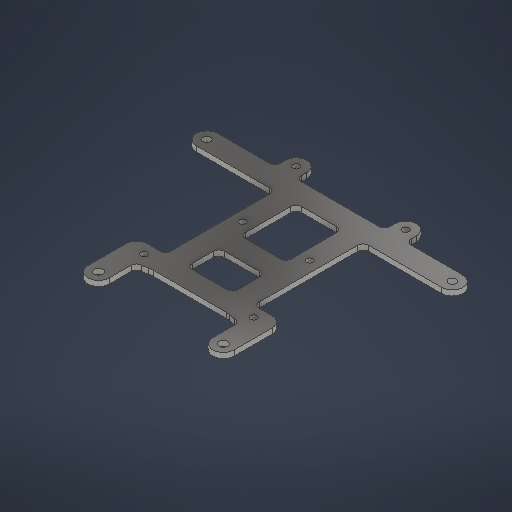
# Autodesk Inventor part: Trägerblech
Saved by Autodesk Inventor 2025.2 (Build 292293000, 293)
## iProperties
Created: 2024-12-09
Part Number: Trägerblech
Material: Generisch
Document SubType Name: Modeling
Designer: Fabian
Density: 1 g/cm^3
Appearance: Stahl - poliert
Author: Fabian
Autodesk Inventor part; units mm, degrees
ref_plane "YZ Plane" through (0, 0, 0) normal (1, 0, 0) x (0, 1, 0)
ref_plane "XZ Plane" through (0, 0, 0) normal (0, 1, 0) x (-1, 0, 0)
ref_plane "XY Plane" through (0, 0, 0) normal (0, 0, 1) x (1, 0, 0)
sketch "Skizze1" plane through (0, 0, 0) normal (0, 1, 0) x (-1, 0, 0)
  circle A0 centre (30.623, -39.877) radius 2.1
  circle A1 centre (30.623, -39.877) radius 2.1
  circle A2 centre (46, -38.5) radius 1.85
  circle A3 centre (46, -38.5) radius 1.85
  circle A4 centre (-30.623, -39.877) radius 2.1
  circle A5 centre (-30.623, -39.877) radius 2.1
  circle A6 centre (-46, -38.5) radius 1.85
  circle A7 centre (-46, -38.5) radius 1.85
  circle A8 centre (-46, 19.5) radius 1.85
  circle A9 centre (-46, 19.5) radius 1.85
  circle A10 centre (-30.1839, 17.0814) radius 2.1
  circle A11 centre (-30.1839, 17.0814) radius 2.1
  circle A12 centre (30.1839, 17.0814) radius 2.1
  circle A13 centre (30.1839, 17.0814) radius 2.1
  circle A14 centre (46, 19.5) radius 1.85
  circle A15 centre (46, 19.5) radius 1.85
  circle A16 centre (23.4, 24.7201) radius 1.2779
  circle A17 centre (-23.4, 24.7201) radius 1.25
  arc A18 (-50, -38.5) -> (-46, -42.5) centre (-46, -38.5) ccw
  line L0 (-50, -38.5) -> (-50, 32.5)
  arc A19 (-46, 36.5) -> (-50, 32.5) centre (-46, 32.5) ccw
  line L1 (-46, 36.5) -> (46, 36.5)
  arc A20 (50, 32.5) -> (46, 36.5) centre (46, 32.5) ccw
  line L2 (50, 32.5) -> (50, -38.5)
  arc A21 (46, -42.5) -> (50, -38.5) centre (46, -38.5) ccw
  line L3 (46, -42.5) -> (36.4, -42.5)
  arc A22 (32.4, -38.5) -> (36.4, -42.5) centre (36.4, -38.5) ccw
  line L4 (32.4, -38.5) -> (32.4, -3.51)
  arc A23 (32.4, -3.51) -> (30.4, -1.51) centre (30.4, -3.51) ccw
  line L5 (30.4, -1.51) -> (-26.4, -1.51)
  arc A24 (-26.4, -1.51) -> (-28.4, -3.51) centre (-26.4, -3.51) ccw
  line L6 (-28.4, -3.51) -> (-28.4, -38.5)
  arc A25 (-32.4, -42.5) -> (-28.4, -38.5) centre (-32.4, -38.5) ccw
  line L7 (-32.4, -42.5) -> (-46, -42.5)
  circle A26 centre (-46, -38.5) radius 1.375
  circle A27 centre (46, 19.5) radius 1.375
  circle A28 centre (46, -38.5) radius 1.375
  circle A29 centre (-46, 19.5) radius 1.375
  line L8 (50, -42.5) -> (-50, -42.5)
  line L9 (-50, -42.5) -> (-50, 36.5)
  line L10 (-50, 36.5) -> (50, 36.5)
  line L11 (50, 36.5) -> (50, -42.5)
  circle A30 centre (-12.55, 10.5) radius 1
  circle A31 centre (-0.05, 10.5) radius 1
  circle A32 centre (-0.05, -10.5) radius 1
  circle A33 centre (-12.55, -10.5) radius 1
  line L12 (-12.55, 12.5) -> (7.45, 12.5)
  arc A34 (9.45, 10.5) -> (7.45, 12.5) centre (7.45, 10.5) ccw
  line L13 (9.45, 10.5) -> (9.45, -10.5)
  arc A35 (7.45, -12.5) -> (9.45, -10.5) centre (7.45, -10.5) ccw
  line L14 (7.45, -12.5) -> (-12.55, -12.5)
  arc A36 (-14.55, -10.5) -> (-12.55, -12.5) centre (-12.55, -10.5) ccw
  line L15 (-14.55, -10.5) -> (-14.55, 10.5)
  arc A37 (-12.55, 12.5) -> (-14.55, 10.5) centre (-12.55, 10.5) ccw
  line L16 (4.8641, 52.5092) -> (13.75, 52.5092)
  arc A38 (19.2723, 46.9869) -> (13.75, 52.5092) centre (13.75, 46.9869) ccw
  line L17 (19.2723, 46.9869) -> (19.2723, 29.5841)
  ellipse E0 centre (20.2732, 29.5863) end of major axis (19.6049, 28.8395) minor radius 1 (19.2723, 29.5841) -> (20.1839, 28.5889) ccw
  line L18 (20.1839, 28.5889) -> (23.7114, 28.2803)
  arc A39 (23.7114, 21.1599) -> (23.7114, 28.2803) centre (23.4, 24.7201) ccw
  line L19 (23.7114, 21.1599) -> (20.1839, 20.8513)
  ellipse E1 centre (20.2732, 19.8539) end of major axis (19.6049, 20.6006) minor radius 1 (20.1839, 20.8513) -> (19.2723, 19.856) ccw
  line L20 (19.2723, 19.856) -> (19.2723, 19.487)
  arc A40 (13.75, 13.9647) -> (19.2723, 19.487) centre (13.75, 19.487) ccw
  line L21 (13.75, 13.9647) -> (-13.75, 13.9647)
  arc A41 (-19.2723, 19.487) -> (-13.75, 13.9647) centre (-13.75, 19.487) ccw
  line L22 (-19.2723, 19.487) -> (-19.2723, 19.856)
  ellipse E2 centre (-20.2732, 19.8539) end of major axis (-19.6049, 20.6006) minor radius 1 (-19.2723, 19.856) -> (-20.1839, 20.8513) ccw
  line L23 (-20.1839, 20.8513) -> (-23.7114, 21.1599)
  arc A42 (-23.7114, 28.2803) -> (-23.7114, 21.1599) centre (-23.4, 24.7201) ccw
  line L24 (-23.7114, 28.2803) -> (-20.1839, 28.5889)
  ellipse E3 centre (-20.2732, 29.5863) end of major axis (-19.6049, 28.8395) minor radius 1 (-20.1839, 28.5889) -> (-19.2723, 29.5841) ccw
  line L25 (-19.2723, 29.5841) -> (-19.2723, 46.9869)
  arc A43 (-13.75, 52.5092) -> (-19.2723, 46.9869) centre (-13.75, 46.9869) ccw
  line L26 (-13.75, 52.5092) -> (-4.8641, 52.5092)
  ellipse E4 centre (-4.8662, 53.5102) end of major axis (-4.1194, 52.8419) minor radius 1 (-4.8641, 52.5092) -> (-3.8688, 53.4208) ccw
  line L27 (-3.8688, 53.4208) -> (-3.5602, 56.9484)
  arc A44 (3.5602, 56.9484) -> (-3.5602, 56.9484) centre (0, 56.6369) ccw
  line L28 (3.5602, 56.9484) -> (3.8688, 53.4208)
  ellipse E5 centre (4.8662, 53.5102) end of major axis (4.1194, 52.8419) minor radius 1 (3.8688, 53.4208) -> (4.8641, 52.5092) ccw
  line L29 (-12.55, -14.5) -> (7.45, -14.5)
  arc A45 (7.45, -14.5) -> (11.45, -10.5) centre (7.45, -10.5) ccw
  line L30 (11.45, -10.5) -> (11.45, 10.5)
  arc A46 (11.45, 10.5) -> (7.45, 14.5) centre (7.45, 10.5) ccw
  line L31 (7.45, 14.5) -> (-12.55, 14.5)
  arc A47 (-12.55, 14.5) -> (-16.55, 10.5) centre (-12.55, 10.5) ccw
  line L32 (-16.55, 10.5) -> (-16.55, -10.5)
  arc A48 (-16.55, -10.5) -> (-12.55, -14.5) centre (-12.55, -10.5) ccw
  line L33 (-12.55, -12.7) -> (7.45, -12.7)
  arc A49 (7.45, -12.7) -> (9.65, -10.5) centre (7.45, -10.5) ccw
  line L34 (9.65, -10.5) -> (9.65, 10.5)
  arc A50 (9.65, 10.5) -> (7.45, 12.7) centre (7.45, 10.5) ccw
  line L35 (7.45, 12.7) -> (-12.55, 12.7)
  arc A51 (-12.55, 12.7) -> (-14.75, 10.5) centre (-12.55, 10.5) ccw
  line L36 (-14.75, 10.5) -> (-14.75, -10.5)
  arc A52 (-14.75, -10.5) -> (-12.55, -12.7) centre (-12.55, -10.5) ccw
  line L37 (16.55, 14.5) -> (-16.55, 14.5)
  line L38 (-16.55, 14.5) -> (-16.55, -14.5)
  line L39 (-16.55, -14.5) -> (16.55, -14.5)
  line L40 (16.55, -14.5) -> (16.55, 14.5)
  line L41 (16.55, 14.5) -> (-16.55, -14.5) construction
  line L42 (-16.55, 14.5) -> (16.55, -14.5) construction
  line L43 (16.55, -14.5) -> (8.55, -14.5)
  line L44 (12.55, -14.5) -> (12.55, -9.5)
  line L45 (16.55, 14.5) -> (16.55, 6.5)
  line L46 (16.55, 10.5) -> (12.55, 10.5)
  line L47 (23.4, 24.7201) -> (23.4, 10.5)
  line L48 (12.55, 10.5) -> (23.4, 10.5) construction
  line L49 (12.55, 14.5) -> (23.4, 14.5)
  line L50 (23.4, 6.5) -> (12.55, 6.5)
  arc A53 (12.55, 14.5) -> (12.55, 6.5) centre (12.55, 10.5) ccw
  arc A54 (23.4, 6.5) -> (23.4, 14.5) centre (23.4, 10.5) ccw
  line L51 (23.4, 10.5) -> (23.4, 24.7201) construction
  line L52 (19.4, 10.5) -> (19.4, 24.7201)
  line L53 (27.4, 24.7201) -> (27.4, 10.5)
  arc A55 (19.4, 10.5) -> (27.4, 10.5) centre (23.4, 10.5) ccw
  arc A56 (27.4, 24.7201) -> (19.4, 24.7201) centre (23.4, 24.7201) ccw
  line L54 (0, -14.5) -> (0, 12.7) construction
  line L55 (12.55, -9.5) -> (12.55, -38.5) construction
  line L56 (8.55, -9.5) -> (8.55, -38.5)
  line L57 (16.55, -38.5) -> (16.55, -9.5)
  arc A57 (16.55, -9.5) -> (8.55, -9.5) centre (12.55, -9.5) ccw
  arc A58 (8.55, -38.5) -> (16.55, -38.5) centre (12.55, -38.5) ccw
  line L58 (12.55, -38.5) -> (46, -38.5) construction
  line L59 (12.55, -42.5) -> (46, -42.5)
  line L60 (46, -34.5) -> (12.55, -34.5)
  arc A59 (12.55, -34.5) -> (12.55, -42.5) centre (12.55, -38.5) ccw
  arc A60 (46, -42.5) -> (46, -34.5) centre (46, -38.5) ccw
  line L61 (-16.55, -14.5) -> (-8.55, -14.5)
  line L62 (-12.55, -14.5) -> (-12.55, -9.5)
  line L63 (-16.55, 14.5) -> (-16.55, 6.5)
  line L64 (-16.55, 10.5) -> (-12.55, 10.5)
  line L65 (-12.55, 10.5) -> (-23.4, 10.5) construction
  line L66 (-12.55, -9.5) -> (-12.55, -38.5) construction
  line L67 (-12.55, -9.5) -> (-12.55, -38.5) construction
  line L68 (-16.55, -9.5) -> (-16.55, -38.5)
  line L69 (-8.55, -38.5) -> (-8.55, -9.5)
  arc A61 (-8.55, -9.5) -> (-16.55, -9.5) centre (-12.55, -9.5) ccw
  arc A62 (-16.55, -38.5) -> (-8.55, -38.5) centre (-12.55, -38.5) ccw
  line L70 (-12.55, 10.5) -> (-23.4, 10.5) construction
  line L71 (-12.55, 14.5) -> (-23.4, 14.5)
  line L72 (-23.4, 6.5) -> (-12.55, 6.5)
  arc A63 (-12.55, 6.5) -> (-12.55, 14.5) centre (-12.55, 10.5) ccw
  arc A64 (-23.4, 14.5) -> (-23.4, 6.5) centre (-23.4, 10.5) ccw
  line L73 (-23.4, 24.7201) -> (-23.4, 10.5) construction
  line L74 (-27.4, 24.7201) -> (-27.4, 10.5)
  line L75 (-19.4, 10.5) -> (-19.4, 24.7201)
  arc A65 (-19.4, 24.7201) -> (-27.4, 24.7201) centre (-23.4, 24.7201) ccw
  arc A66 (-27.4, 10.5) -> (-19.4, 10.5) centre (-23.4, 10.5) ccw
  line L76 (12.55, -9.5) -> (12.55, 10.5) construction
  line L77 (16.55, -9.5) -> (16.55, 10.5)
  line L78 (8.55, 10.5) -> (8.55, -9.5)
  arc A67 (8.55, -9.5) -> (16.55, -9.5) centre (12.55, -9.5) ccw
  arc A68 (16.55, 10.5) -> (8.55, 10.5) centre (12.55, 10.5) ccw
  line L79 (-12.55, -10.5) -> (-12.55, 10.5) construction
  line L80 (-16.55, -10.5) -> (-16.55, 10.5)
  line L81 (-8.55, 10.5) -> (-8.55, -10.5)
  arc A69 (-16.55, -10.5) -> (-8.55, -10.5) centre (-12.55, -10.5) ccw
  arc A70 (-8.55, 10.5) -> (-16.55, 10.5) centre (-12.55, 10.5) ccw
  line L82 (-12.55, 10.5) -> (12.55, 10.5) construction
  line L83 (-12.55, 14.5) -> (12.55, 14.5)
  line L84 (12.55, 6.5) -> (-12.55, 6.5)
  arc A71 (-12.55, 14.5) -> (-12.55, 6.5) centre (-12.55, 10.5) ccw
  arc A72 (12.55, 6.5) -> (12.55, 14.5) centre (12.55, 10.5) ccw
  line L85 (12.55, -9.5) -> (-12.55, -9.5) construction
  line L86 (12.55, -5.5) -> (-12.55, -5.5)
  line L87 (-12.55, -13.5) -> (12.55, -13.5)
  arc A73 (12.55, -13.5) -> (12.55, -5.5) centre (12.55, -9.5) ccw
  arc A74 (-12.55, -5.5) -> (-12.55, -13.5) centre (-12.55, -9.5) ccw
  line L88 (-46, -38.5) -> (-12.55, -38.5) construction
  line L89 (-46, -34.5) -> (-12.55, -34.5)
  line L90 (-12.55, -42.5) -> (-46, -42.5)
  arc A75 (-46, -34.5) -> (-46, -42.5) centre (-46, -38.5) ccw
  arc A76 (-12.55, -42.5) -> (-12.55, -34.5) centre (-12.55, -38.5) ccw
  line L91 (-12.55, -38.5) -> (12.55, -38.5) construction
  line L92 (-12.55, -34.5) -> (12.55, -34.5)
  line L93 (12.55, -42.5) -> (-12.55, -42.5)
  arc A77 (-12.55, -34.5) -> (-12.55, -42.5) centre (-12.55, -38.5) ccw
  arc A78 (12.55, -42.5) -> (12.55, -34.5) centre (12.55, -38.5) ccw
  circle A79 centre (23.4, 24.7201) radius 1.6
  circle A80 centre (-23.4, 24.7201) radius 1.6
  circle A81 centre (46, -38.5) radius 1.45
  circle A82 centre (-46, -38.5) radius 1.45
  point P0 (0, 0)
  point P1 (0, 0)
  point P2 (366.8028, -91.5166)
  point P3 (345.2028, -91.5166)
  point P4 (266.8028, -155.8292)
  point P5 (266.8028, -165.2628)
  point P6 (366.8028, -165.2628)
  point P7 (366.8028, -155.8292)
  point P8 (284.4028, -91.5166)
  point P9 (266.8028, -170.5166)
  point P10 (366.8028, -170.5166)
  point P11 (366.8028, -155.8285)
  point P12 (345.2028, -91.5166)
  point P13 (366.8028, -155.8285)
  point P14 (366.8028, -155.8292)
  point P15 (266.8028, -155.8285)
  point P16 (266.8028, -91.5166)
  point P17 (284.4028, -91.5166)
  point P18 (266.8028, -155.8285)
  point P19 (266.8028, -155.8292)
  point P20 (0, 0)
  point P21 (0, 31.237)
  point P22 (17.975, 10.5)
  point P23 (23.4, 17.61)
  point P24 (12.55, -24)
  point P25 (29.275, -38.5)
  point P26 (-12.55, -24)
  point P27 (-17.975, 10.5)
  point P28 (-23.4, 17.61)
  point P29 (12.55, 0.5)
  point P30 (-12.55, 0)
  point P31 (0, 10.5)
  point P32 (0, -9.5)
  point P33 (-29.275, -38.5)
  point P34 (0, -38.5)
  point P35 (19.4, 14.5)
  point P36 (7.45, 14.5)
  point P37 (-19.4, 14.5)
  point P38 (-16.55, -34.5)
  point P39 (-50, -38.5)
  point P40 (-32.4, -42.5)
  point P41 (16.55, -34.5)
  point P42 (8.55, -13.5)
  point P43 (8.55, -34.5)
  point P44 (-8.55, -34.5)
  point P45 (-8.55, -13.5)
  point P46 (8.55, -5.5)
  point P47 (-8.55, -5.5)
  point P48 (-8.55, 6.5)
  point P49 (8.55, 6.5)
  point P50 (16.1218, 14.5)
  point P51 (-16.1218, 14.5)
  dimension "d5" = 2
  dimension "d6" = 0.2
  dimension "d7" = 8
  dimension "d8" = 5
  dimension "d9" = 8
  dimension "d10" = 4
  dimension "d11" = 8
  dimension "d12" = 8
  dimension "d13" = 8
  dimension "d14" = 8
  dimension "d15" = 8
  dimension "d19" = 3.2
  dimension "d20" = 3.2
  dimension "d69" = 2.9
  dimension "d70" = 2.9
  constraints: 218 end point, 106 point on circle, 83 centre point, 53 tangent, 20 parallel, 18 midpoint, 12 coincident, 6 perpendicular, 6 point on line, 6 symmetric about line, 5 horizontal, 3 collinear, 3 vertical, 2 concentric, 38 other
  measures "d5" distance between parallel lines of L14 L29
  measures "d6" distance between parallel lines of L14 L33
  measures "d7" distance of L39.end L43.end
  measures "d8" distance of L44.start L44.end
  measures "d9" distance of L37.start L45.end
  measures "d10" distance of L46.start L46.end
  measures "d11" diameter of A58
  measures "d12" diameter of A60
  measures "d13" diameter of A62
  measures "d14" diameter of A64
  measures "d15" diameter of A66
  measures "d19" diameter of A79
  measures "d20" diameter of A80
  measures "d69" diameter of A81
  measures "d70" diameter of A82
extrude "Extrusion1" add sketch "Skizze1" along normal blind 2 contours A0 A22 | A0 A22 L4 L60 A60 A21 L3 | A22 A0 | A0 A22 L8 A58 L57 L60 L4 | L8 A62 L69 L92 L56 A58 | A58 A59 A78 | L60 L92 L56 L39 L57 | L57 A78 L60 | L8 A25 A4 L6 L89 L68 A62 | A62 A77 A76 | L56 L92 A59 | L39 L44 A67 L40 | L7 A18 A75 L89 L6 A25 A4 | L68 L89 A77 | A76 L92 L69 | L40 A57 L86 L30 L5 | L5 L30 L84 L50 L40 | L39 L56 A45 L87 L44 | A67 A45 L30 A57 | A25 A4 | A4 A25 | L68 L39 L29 L69 L92 L89 | L30 L86 L34 L5 | L5 L34 L84 L30 | L50 A72 L40 | L40 L49 L52 A55 L50 | L87 A45 A67 | A57 L30 L86 | L38 A48 L39 | L29 A69 L87 L69 | L56 L87 A45 | L34 L86 L13 L5 | L5 L13 L84 L34 | L30 A57 L34 L86 | L84 L34 A53 L30 | L30 A53 L84 | A68 A40 L37 L40 | A72 A53 L30 A46 L21 A40 A68 | A55 L52 L49 A54 | A67 A49 L34 A57 L30 A45 | A45 L87 L56 A49 A67 | L32 A74 L62 A48 | L62 L87 A69 | L87 A69 L33 L69 | L69 L33 A49 L56 L87 | L13 L86 L78 L5 | L5 L78 L84 L13 | L34 A57 L13 L86 | L84 L13 A53 L34 | A53 L34 A50 A46 L30 | A54 L47 L19 A39 L18 A56 L53 | A67 A35 L13 A57 L34 A49 | A49 L56 A35 A67 | L32 L5 L36 A61 | A61 L36 A52 L62 A74 | L62 L33 A69 L87 | L69 L14 A35 L56 A49 L33 | L33 A69 L14 L69 | L84 L78 A53 L13 | L13 A57 L78 L86 | A53 L13 A34 A50 L34 | L52 E1 L19 L47 L49 | A67 A57 L13 A35 | A35 L56 A67 | L18 A39 L19 E1 L52 A56 | L32 L72 L36 L5 | A61 L15 A36 L62 A52 L36 | L36 L5 L15 A61 | L62 L14 A69 L33 | L69 L81 L86 L78 L56 A35 L14 | L14 A69 L69 | L81 L86 A61 L15 L5 | L5 L15 L72 L84 L81 | L84 L81 A63 L12 A34 A53 L78 | A53 A34 L13 | A53 A50 L35 A63 L21 A46 | A46 L21 A53 | A65 L75 E2 L23 A42 L24 | L24 A42 L23 E2 L75 L71 A64 L74 A65 | L36 L72 L15 L5 | L72 A66 L75 L71 L38 L32 | L32 A71 L36 L72 | A61 L69 A69 L14 A36 L15 | L84 A63 L81 | L81 A61 L86 | A53 A34 L12 A63 L35 A50 | L36 A71 L15 L72 | L38 L37 A41 A47 | A47 A41 L21 A63 L35 A51 L64 | L64 L36 A71 | A64 L71 L75 A66 | L15 A71 L72 | A63 A71 L15 A37 L12 | L36 L64 L15 A71 | A51 L35 A63 L12 A37 L64 | A2 | A6 | A30 | A31 | A32 | A33 L62 | L62 A33
fillet "Rundung1" radius 2 14 edges at (-16.55, 1, -34.5) (-8.55, 1, -34.5) (8.55, 1, -34.5) (16.55, 1, -34.5) (8.55, 1, -13.5) (-8.55, 1, -13.5) (-8.55, 1, -5.5) (8.55, 1, -5.5) (8.55, 1, 6.5) (-8.55, 1, 6.5) (-19.4, 1, 14.5) (-16.55, 1, 6.5) (16.55, 1, 6.5) (19.4, 1, 14.5)
fillet "Rundung2" radius 8 2 edges at (16.1218, 1, 14.5) (-16.1218, 1, 14.5)
sketch "Skizze4" plane through (0, 2, 0) normal (0, 1, 0) x (1, 0, 0)
  line L0 (20.55, 10.5) -> (-20.55, 10.5)
  line L1 (-20.55, 10.5) -> (-20.55, -10.5)
  line L2 (-20.55, -10.5) -> (20.55, -10.5)
  line L3 (20.55, -10.5) -> (20.55, 10.5)
  line L4 (20.55, 10.5) -> (-20.55, -10.5) construction
  line L5 (-20.55, 10.5) -> (20.55, -10.5) construction
  line L6 (-20.55, 10.5) -> (-20.55, 42.5)
  line L7 (-20.55, 42.5) -> (-20.55, 46.5)
  line L8 (0, 10.5) -> (0, -10.5) construction
  line L9 (20.55, 10.5) -> (20.55, 42.5) construction
  line L10 (20.55, 42.5) -> (20.55, 46.5) construction
  circle A0 centre (-20.55, -10.5) radius 1.2295 construction
  circle A1 centre (20.55, -10.5) radius 1.2295 construction
  line L11 (0, 10.5) -> (0, 18.5) construction
  line L12 (0, 18.5) -> (-12.55, 18.5) construction
  line L13 (0, 18.5) -> (12.55, 18.5) construction
  point P0 (0, 0)
  dimension "d45" = 41.1
  dimension "d46" = 32
  dimension "d47" = 4
  dimension "d48" = 41.1
  dimension "d49" = 10.5
  dimension "d50" = 32
  dimension "d51" = 4
  dimension "d52" = 8
  dimension "d53" = 12.55
  dimension "d54" = 12.55
  constraints: 28 end point, 6 coincident, 4 midpoint, 4 vertical, 3 horizontal, 2 parallel, 1 perpendicular, 1 point on line
  measures "d45" distance of L0.start L0.end
  measures "d46" distance of L0.end L6.end
  measures "d47" distance of L6.end L7.end
  measures "d48" distance between parallel lines of L6 L3
  measures "d49" distance from line of point (0, 0) L0
  measures "d50" distance of L0.start L9.end
  measures "d51" distance of L9.end L10.end
  measures "d52" distance of L8.start L11.end
  measures "d53" distance of L11.end L12.end
  measures "d54" distance of L11.end L13.end
sketch "Skizze5" plane through (0, 2, 0) normal (0, 1, 0) x (1, 0, 0)
  line L0 (0, 0) -> (-20.55, 0)
  line L1 (-20.55, 0) -> (-20.55, 46.5)
  line L2 (-20.55, 46.5) -> (-20.55, 42.5) construction
  line L3 (-24.55, 46.5) -> (-24.55, 42.5)
  line L4 (-16.55, 42.5) -> (-16.55, 46.5)
  arc A0 (-16.55, 46.5) -> (-24.55, 46.5) centre (-20.55, 46.5) ccw
  arc A1 (-24.55, 42.5) -> (-16.55, 42.5) centre (-20.55, 42.5) ccw
  line L5 (0, 0) -> (0, 2.0706)
  line L6 (24.55, 46.5) -> (24.55, 42.5)
  line L7 (16.55, 42.5) -> (16.55, 46.5)
  arc A2 (24.55, 46.5) -> (16.55, 46.5) centre (20.55, 46.5) ccw
  line L8 (-24.55, 42.5) -> (24.55, 42.5)
  point P0 (-20.55, 44.5)
  dimension "d55" = 20.55
  dimension "d56" = 46.5
  dimension "d57" = 4
  dimension "d58" = 8
  constraints: 20 end point, 6 point on circle, 5 symmetric about line, 4 tangent, 3 centre point, 2 horizontal, 1 midpoint, 1 parallel, 1 perpendicular, 1 point on line, 1 vertical, 1 other
  measures "d55" distance of L0.start L0.end
  measures "d56" distance of L0.end L1.end
  measures "d57" distance of L1.end L2.end
  measures "d58" diameter of A1
extrude "Extrusion3" add sketch "Skizze5" against normal up to surface (2 mm away) contours L8 L3 A0 L4 | L6 L8 L7 A2
hole "Bohrung2" at (-20.55, 2, -46.5) at (20.55, 2, -46.5) at (-20.55, 2, 10.5) at (20.55, 2, 10.5) at (-12.55, 2, -18.5) at (12.55, 2, -18.5) direction (0, -1, 0) diameter 2.459 depth 8.8 tip angle 118 thread size "M3x0.5" class "6H" standard "ISO Metric profile"
fillet "Rundung3" radius 2 4 edges at (-16.55, 1, -42.5) (-24.55, 1, -42.5) (16.55, 1, -42.5) (24.55, 1, -42.5)
